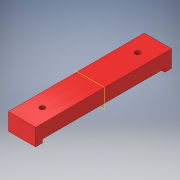
# Autodesk Inventor part: BandSawJigTop
Saved by Autodesk Inventor 2018.2 (Build 222227000, 227)
## iProperties
Created: 2017-12-10
Part Number: BandSawJigTop
Material: LCP Plastic
Document SubType Name: Modeling
Designer: steele
Density: 1.626 g/cm^3
Appearance: Light Red
Author: steele
Autodesk Inventor part; units mm, degrees
ref_plane "YZ Plane" through (0, 0, 0) normal (1, 0, 0) x (0, 1, 0)
ref_plane "XZ Plane" through (0, 0, 0) normal (0, 1, 0) x (-1, 0, 0)
sketch "Sketch1" plane through (0, 0, 0) normal (0, 1, 0) x (-1, 0, 0)
  line L0 (25.4, 127) -> (-25.4, 127)
  line L1 (-25.4, 127) -> (-25.4, -127)
  line L2 (-25.4, -127) -> (25.4, -127)
  line L3 (25.4, -127) -> (25.4, 127)
  line L4 (25.4, 127) -> (-25.4, -127) construction
  line L5 (-25.4, 127) -> (25.4, -127) construction
  point P0 (0, 0)
  dimension "d0" = 50.8
  dimension "d1" = 254
  constraints: 12 end point, 2 midpoint, 2 parallel, 1 horizontal, 1 perpendicular
  measures "d0" distance of L0.start L0.end
  measures "d1" distance of L1.end L0.end
extrude "Extrusion1" add sketch "Sketch1" along normal blind 25.4
sketch "Sketch2" plane through (0, 0, 0) normal (0, -1, 0) x (1, 0, 0)
  line L0 (-25.4, 127) -> (-25.4, 114.3)
  line L1 (-25.4, 114.3) -> (25.4, 114.3)
  line L2 (25.4, 114.3) -> (25.4, 127)
  line L3 (25.4, 127) -> (-25.4, 127)
  line L4 (-25.4, 127) -> (25.4, 114.3) construction
  line L5 (-25.4, 114.3) -> (25.4, 127) construction
  line L6 (-25.4, 127) -> (25.4, 127) projected
  point P0 (0, 0)
  point P1 (0, 120.65)
  dimension "d4" = 12.7
  dimension "d5" = 25.4
  dimension "d6" = 0
  constraints: 12 end point, 2 midpoint, 2 parallel, 1 perpendicular, 1 vertical
  measures "d4" distance of L0.start L0.end
  measures "d5" distance from line of L0 point (0, 120.65)
  measures "d6" distance between parallel lines of L6 L3
extrude "Extrusion2" add sketch "Sketch2" along normal blind 6.35
mirror "Mirror1" about plane through (0, 0, 0) normal (0, 0, 1) of "Extrusion2"
sketch "Sketch3" plane through (0, 25.4, 0) normal (0, 1, 0) x (1, 0, 0)
  circle A0 centre (0, -88.9) radius 4.7625
  line L0 (-25.4, -127) -> (25.4, -127) projected
  point P0 (0, 0)
  dimension "d9" = 9.525
  dimension "d10" = 38.1
  constraints: 1 centre point
  measures "d9" diameter of A0
  measures "d10" distance from line of A0.centre L0
extrude "Extrusion3" cut sketch "Sketch3" against normal through all
mirror "Mirror2" about plane through (0, 0, 0) normal (0, 0, 1) of "Extrusion3"
body "Solid1"
